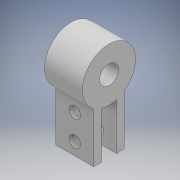
# Autodesk Inventor part: servo attachment
Saved by Autodesk Inventor 2017 (Build 210142000, 142)
## iProperties
Created: 2017-04-28
Part Number: servo attachment
Material: Generic
Document SubType Name: Modeling
Designer: s4321966
Density: 1 g/cm^3
Appearance: Default
Author: s4321966
Autodesk Inventor part; units mm, degrees
ref_plane "YZ Plane" through (0, 0, 0) normal (1, 0, 0) x (0, 1, 0)
ref_plane "XZ Plane" through (0, 0, 0) normal (0, 1, 0) x (-1, 0, 0)
ref_plane "XY Plane" through (0, 0, 0) normal (0, 0, 1) x (1, 0, 0)
sketch "Sketch1" plane through (0, 0, 0) normal (1, 0, 0) x (0, 1, 0)
  circle A0 centre (0, 0) radius 3.5
  circle A1 centre (0, 0) radius 1.25
  line L0 (0, -3.5) -> (1, -3.5)
  line L1 (1, -3.5) -> (1, -9.5)
  line L2 (1, -9.5) -> (0, -9.5)
  line L3 (0, -9.5) -> (0, -3.5)
  line L4 (1, -9.5) -> (2.0279, -9.5)
  line L5 (2.0279, -9.5) -> (2.0279, -1.25)
  line L6 (2.0279, -1.25) -> (1, -1.25)
  line L7 (1, -1.25) -> (1, -9.5)
  line L8 (0, -3.5) -> (-1, -3.5)
  line L9 (-1, -3.5) -> (-1, -9.5)
  line L10 (-1, -9.5) -> (0, -9.5)
  line L11 (-1, -9.5) -> (-2.0279, -9.5)
  line L12 (-2.0279, -9.5) -> (-2.0279, -1.25)
  line L13 (-2.0279, -1.25) -> (-1, -1.25)
  line L14 (-1, -1.25) -> (-1, -9.5)
  dimension "d0" = 7
  dimension "d1" = 2.5
  dimension "d2" = 1
  dimension "d3" = 6
  constraints: 30 end point, 5 symmetric about line, 4 coincident, 4 parallel, 2 horizontal, 2 perpendicular, 1 centre point, 1 vertical alignment, 2 other
  measures "d1" diameter of A1
  measures "d2" distance of L1.end L2.end
  measures "d3" distance of L0.end L1.end
extrude "Extrusion1" add sketch "Sketch1" along normal blind 5 contours A0 L5 L6 L7 L14 L13 L12 | L12 L13 L14 A0 | A0 L14 L9 L11 L12 | L5 L4 L1 L7 A0 | A0 L7 L6 L5
sketch "Sketch2" plane through (0, 2.0279, -2.8527) normal (0, 1, 0) x (1, 0, 0)
  line L0 (0, 6.6473) -> (5, 6.6473) projected
  line L1 (2.5, 6.6473) -> (2.5, 0)
  line L2 (5, 0) -> (0, 0) projected
  line L3 (2.5, 3.3237) -> (0, 6.6473)
  line L4 (0, 6.6473) -> (5.0696, 3.3237)
  line L5 (5.0696, 3.3237) -> (0, 0)
  circle A0 centre (2.5348, 1.6618) radius 0.75
  circle A1 centre (2.5348, 4.9855) radius 0.75
  point P0 (0, -2.8527)
  dimension "d6" = 1.5
  dimension "d7" = 1.5
  constraints: 8 end point, 5 midpoint, 2 centre point
  measures "d6" diameter of A0
  measures "d7" diameter of A1
extrude "Extrusion2" cut sketch "Sketch2" against normal blind 5 contours A1 L1 L4 | L4 L1 A1 | A1 L4 L1 | L1 L4 A1 | A0 L5 L1 | L1 L5 A0 | L5 A0 L1 | L1 A0 L5
body "Solid1"
